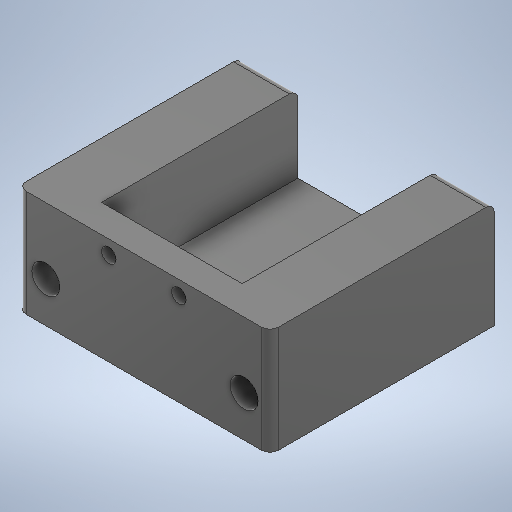
# Autodesk Inventor part: T-Frame_encoder_frame
Saved by Autodesk Inventor 2026.2 (Build 302298010, 298A)
## iProperties
Created: 2026-05-20
Part Number: T-Frame_encoder_frame
Material: ABS Plastic
Document SubType Name: Modeling
Designer: chanh
Density: 1.06 g/cm^3
Appearance: Smooth - White
Author: chanh
Autodesk Inventor part; units mm, degrees
ref_plane "YZ Plane" through (0, 0, 0) normal (1, 0, 0) x (0, 1, 0)
ref_plane "XZ Plane" through (0, 0, 0) normal (0, 1, 0) x (-1, 0, 0)
ref_plane "XY Plane" through (0, 0, 0) normal (0, 0, 1) x (1, 0, 0)
sketch "Sketch1" plane through (0, 0, 0) normal (0, 1, 0) x (-1, 0, 0)
  line L0 (45, -40) -> (-45, -40)
  line L1 (-45, -40) -> (-45, 40)
  line L2 (-45, 40) -> (45, 40)
  line L3 (45, 40) -> (45, -40)
  line L4 (45, -40) -> (-45, 40) construction
  line L5 (-45, -40) -> (45, 40) construction
  point P0 (0, 0)
  dimension "d0" = 90
  dimension "d1" = 80
  constraints: 12 end point, 2 midpoint, 2 parallel, 1 horizontal, 1 perpendicular
  measures "d0" distance of L0.start L0.end
  measures "d1" distance of L0.end L1.end
extrude "Extrusion1" add sketch "Sketch1" along normal blind 38
sketch "Sketch2" plane through (0, 38, 0) normal (0, 1, 0) x (1, 0, 0)
  line L0 (-45, -40) -> (45, -40) projected
  line L1 (45, -40) -> (45, 40) projected
  line L2 (45, 40) -> (-45, 40) projected
  line L3 (-45, 40) -> (-45, -40) projected
  line L4 (-25.1, 40) -> (25.1, 40)
  line L5 (25.1, 40) -> (25.1, 20)
  line L6 (25.1, 20) -> (-25.1, 20)
  line L7 (-25.1, 20) -> (-25.1, 40)
  line L8 (-25.1, 20) -> (25.1, 20)
  line L9 (25.1, 20) -> (25.1, -30)
  line L10 (25.1, -30) -> (-25.1, -30)
  line L11 (-25.1, -30) -> (-25.1, 20)
  point P0 (0, 0)
  point P1 (0, 40)
  dimension "d4" = 50.2
  dimension "d5" = 20
  dimension "d24" = 50
  constraints: 16 end point, 4 parallel, 2 horizontal, 2 midpoint, 2 perpendicular, 1 collinear, 1 point on line
  measures "d4" distance of L9.end L10.end
  measures "d5" distance between parallel lines of L2 L6
  measures "d24" distance between parallel lines of L6 L10
extrude "Extrusion2" cut sketch "Sketch2" against normal blind 27.5 contours L2 L5 L6 L7 | L6 L9 L10 L11
sketch "Sketch3" plane through (-45, 0, 40) normal (0, 0, 1) x (1, 0, 0)
  circle A0 centre (32.5, 33) radius 2.067 construction
  circle A1 centre (57.5, 33) radius 2.067 construction
  line L0 (0, 0) -> (90, 0) construction
  line L1 (90, 0) -> (90, 38) construction
  line L2 (0, 38) -> (90, 38) construction
  line L3 (0, 0) -> (0, 38) construction
  line L4 (0, 15) -> (90, 15) construction
  line L5 (45, 0) -> (45, 38) construction
  point P0 (10, 15)
  point P1 (80, 15)
  dimension "d8" = 15
  dimension "d9" = 10
  constraints: 4 end point, 3 point on line, 2 coincident, 1 midpoint, 1 perpendicular, 1 symmetric about line
  measures "d8" distance between parallel lines of L4 L0
  measures "d9" distance from line of L3 point (10, 15)
hole "Hole1" at (-12.5, 33, 40) at (12.5, 33, 40) direction (0, 0, -1) diameter 5.2 end through all
sketch "Sketch4" plane through (-45, 0, 40) normal (0, 0, 1) x (1, 0, 0)
  point P0 (45, 0)
  point P1 (10.0426, 14.4118)
  point P2 (80.769, 14.5558)
hole "Hole2" at (-34.9574, 14.4118, 40) at (35.769, 14.5558, 40) direction (0, 0, -1) diameter 5.2 end through all counterbore diameter 10 counterbore depth 48
fillet "Fillet1" radius 3 4 edges at (-45, 19, 40) (45, 19, 40) (35.05, 38, -40) (-35.05, 38, -40)
body "Solid1"
